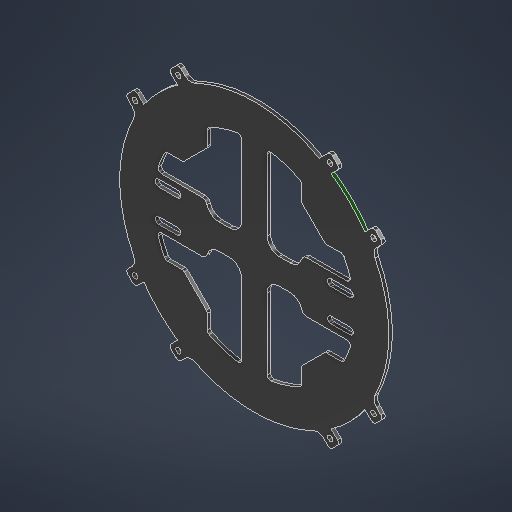
# Autodesk Inventor part: Line Board
Saved by Autodesk Inventor 2026.1 (Build 301233020, 233B)
## iProperties
Created: 2025-11-07
Part Number: Line Board
Material: Generic
Document SubType Name: Modeling
Designer: Bahaa
Density: 1 g/cm^3
Appearance: Glossy - Black
Author: Bahaa
Autodesk Inventor part; units mm, degrees
ref_plane "YZ Plane" through (0, 0, 0) normal (1, 0, 0) x (0, 1, 0)
ref_plane "XZ Plane" through (0, 0, 0) normal (0, 1, 0) x (-1, 0, 0)
ref_plane "XY Plane" through (0, 0, 0) normal (0, 0, 1) x (1, 0, 0)
sketch "Sketch1" plane through (0, 0, 0) normal (0, 1, 0) x (-1, 0, 0)
  circle A0 centre (0, 0) radius 79
  circle A1 centre (0, 0) radius 59
  line L0 (-75, 7.5) -> (75, 7.5)
  line L1 (75, 7.5) -> (75, -7.5)
  line L2 (75, -7.5) -> (-75, -7.5)
  line L3 (-75, -7.5) -> (-75, 7.5)
  line L4 (-75, 7.5) -> (75, -7.5) construction
  line L5 (75, 7.5) -> (-75, -7.5) construction
  line L6 (-7.5, -75) -> (-7.5, 75)
  line L7 (7.5, 75) -> (7.5, -75)
  line L8 (75, -7.5) -> (-75, -7.5)
  line L9 (-75, 7.5) -> (75, 7.5)
  line L10 (7.5, 75) -> (7.5, -75)
  line L11 (-7.5, -75) -> (-7.5, 75)
  line L12 (7.5, 25) -> (-7.5, 25)
  line L13 (-25, 7.5) -> (-25, -7.5)
  line L14 (-7.5, -25) -> (7.5, -25)
  line L15 (25, -7.5) -> (25, 7.5)
  line L16 (25, 25) -> (-25, -25) construction
  line L17 (-25, 25) -> (25, -25) construction
  line L18 (-7.5, 25) -> (-25, 7.5)
  line L19 (25, 7.5) -> (7.5, 25)
  line L20 (25, -7.5) -> (7.5, -25)
  line L21 (-25, -7.5) -> (-7.5, -25)
  line L22 (0, 0) -> (57.2756, -57.2756) construction
  line L23 (57.2756, -57.2756) -> (44.5477, -70.0036) construction
  circle A2 centre (44.5477, -70.0036) radius 1.6
  line L24 (44.5477, -70.0036) -> (47.3762, -67.1751) construction
  line L25 (47.3762, -67.1751) -> (50.2046, -70.0036)
  line L26 (50.2046, -70.0036) -> (44.5477, -64.3467)
  line L27 (44.5477, -64.3467) -> (38.8909, -70.0036) construction
  line L28 (38.8909, -70.0036) -> (44.5477, -75.6604)
  line L29 (44.5477, -75.6604) -> (50.2046, -70.0036)
  line L30 (38.8909, -70.0036) -> (38.0953, -69.208)
  line L31 (44.5477, -64.3467) -> (45.0778, -64.8768)
  circle A3 centre (70.0036, -44.5477) radius 1.6
  line L32 (70.0036, -44.5477) -> (67.1751, -47.3762) construction
  line L33 (67.1751, -47.3762) -> (70.0036, -50.2046)
  line L34 (70.0036, -50.2046) -> (64.3467, -44.5477)
  line L35 (64.3467, -44.5477) -> (70.0036, -38.8909) construction
  line L36 (70.0036, -38.8909) -> (75.6604, -44.5477)
  line L37 (75.6604, -44.5477) -> (70.0036, -50.2046)
  line L38 (70.0036, -38.8909) -> (69.208, -38.0953)
  line L39 (64.3467, -44.5477) -> (64.8768, -45.0778)
  line L40 (64.3467, 44.5477) -> (64.8768, 45.0778)
  line L41 (70.0036, 38.8909) -> (69.208, 38.0953)
  line L42 (64.3467, 44.5477) -> (70.0036, 38.8909) construction
  line L43 (70.0036, 44.5477) -> (67.1751, 47.3762) construction
  circle A4 centre (70.0036, 44.5477) radius 1.6
  line L44 (70.0036, 50.2046) -> (64.3467, 44.5477)
  line L45 (70.0036, 38.8909) -> (75.6604, 44.5477)
  line L46 (75.6604, 44.5477) -> (70.0036, 50.2046)
  line L47 (57.2756, 57.2756) -> (70.0036, 44.5477) construction
  line L48 (67.1751, 47.3762) -> (70.0036, 50.2046)
  line L49 (44.5477, 64.3467) -> (45.0778, 64.8768)
  line L50 (47.3762, 67.1751) -> (50.2046, 70.0036)
  line L51 (50.2046, 70.0036) -> (44.5477, 64.3467)
  line L52 (44.5477, 70.0036) -> (47.3762, 67.1751) construction
  circle A5 centre (44.5477, 70.0036) radius 1.6
  line L53 (44.5477, 75.6604) -> (50.2046, 70.0036)
  line L54 (44.5477, 64.3467) -> (38.8909, 70.0036) construction
  line L55 (38.8909, 70.0036) -> (38.0953, 69.208)
  line L56 (38.8909, 70.0036) -> (44.5477, 75.6604)
  line L57 (-44.5477, 64.3467) -> (-45.0778, 64.8768)
  line L58 (-38.8909, 70.0036) -> (-38.0953, 69.208)
  line L59 (-44.5477, 64.3467) -> (-38.8909, 70.0036) construction
  line L60 (-44.5477, 70.0036) -> (-47.3762, 67.1751) construction
  circle A6 centre (-44.5477, 70.0036) radius 1.6
  line L61 (-50.2046, 70.0036) -> (-44.5477, 64.3467)
  line L62 (-38.8909, 70.0036) -> (-44.5477, 75.6604)
  line L63 (-44.5477, 75.6604) -> (-50.2046, 70.0036)
  line L64 (-57.2756, 57.2756) -> (-44.5477, 70.0036) construction
  line L65 (-47.3762, 67.1751) -> (-50.2046, 70.0036)
  line L66 (-64.3467, 44.5477) -> (-64.8768, 45.0778)
  line L67 (-67.1751, 47.3762) -> (-70.0036, 50.2046)
  line L68 (-70.0036, 50.2046) -> (-64.3467, 44.5477)
  line L69 (-70.0036, 44.5477) -> (-67.1751, 47.3762) construction
  circle A7 centre (-70.0036, 44.5477) radius 1.6
  line L70 (-75.6604, 44.5477) -> (-70.0036, 50.2046)
  line L71 (-64.3467, 44.5477) -> (-70.0036, 38.8909) construction
  line L72 (-70.0036, 38.8909) -> (-69.208, 38.0953)
  line L73 (-70.0036, 38.8909) -> (-75.6604, 44.5477)
  line L74 (-64.3467, -44.5477) -> (-64.8768, -45.0778)
  line L75 (-70.0036, -38.8909) -> (-69.208, -38.0953)
  line L76 (-64.3467, -44.5477) -> (-70.0036, -38.8909) construction
  line L77 (-70.0036, -44.5477) -> (-67.1751, -47.3762) construction
  circle A8 centre (-70.0036, -44.5477) radius 1.6
  line L78 (-70.0036, -50.2046) -> (-64.3467, -44.5477)
  line L79 (-70.0036, -38.8909) -> (-75.6604, -44.5477)
  line L80 (-75.6604, -44.5477) -> (-70.0036, -50.2046)
  line L81 (-57.2756, -57.2756) -> (-70.0036, -44.5477) construction
  line L82 (-67.1751, -47.3762) -> (-70.0036, -50.2046)
  line L83 (-44.5477, -64.3467) -> (-45.0778, -64.8768)
  line L84 (-47.3762, -67.1751) -> (-50.2046, -70.0036)
  line L85 (-50.2046, -70.0036) -> (-44.5477, -64.3467)
  line L86 (-44.5477, -70.0036) -> (-47.3762, -67.1751) construction
  circle A9 centre (-44.5477, -70.0036) radius 1.6
  line L87 (-44.5477, -75.6604) -> (-50.2046, -70.0036)
  line L88 (-44.5477, -64.3467) -> (-38.8909, -70.0036) construction
  line L89 (-38.8909, -70.0036) -> (-38.0953, -69.208)
  line L90 (-38.8909, -70.0036) -> (-44.5477, -75.6604)
  line L91 (55.8614, 55.8614) -> (65.7609, 45.9619) construction
  line L92 (65.7609, 45.9619) -> (65.6902, 45.8912) construction
  line L93 (65.6902, 45.8912) -> (45.8912, 65.6902)
  line L94 (-45.8912, 65.6902) -> (-65.6902, 45.8912)
  line L95 (-65.6902, -45.8912) -> (-45.8912, -65.6902)
  line L96 (45.8912, -65.6902) -> (65.6902, -45.8912)
  line L97 (70.25, -7.5) -> (87.75, -7.5)
  line L98 (87.75, -7.5) -> (87.75, 7.5)
  line L99 (87.75, 7.5) -> (70.25, 7.5)
  line L100 (70.25, 7.5) -> (70.25, -7.5)
  line L101 (70.25, -7.5) -> (87.75, 7.5) construction
  line L102 (87.75, -7.5) -> (70.25, 7.5) construction
  line L103 (0, -7.5) -> (0, 7.5) construction
  line L104 (-70.25, -7.5) -> (-87.75, -7.5)
  line L105 (-87.75, -7.5) -> (-87.75, 7.5)
  line L106 (-87.75, 7.5) -> (-70.25, 7.5)
  line L107 (-70.25, 7.5) -> (-70.25, -7.5)
  line L108 (10, 49) -> (-10, 49)
  line L109 (-10, 49) -> (-10, 59) construction
  line L110 (-10, 59) -> (10, 59) construction
  line L111 (10, 59) -> (10, 49) construction
  line L112 (10, 49) -> (-10, 59) construction
  line L113 (-10, 49) -> (10, 59) construction
  line L114 (10, 49) -> (17.3816, 56.3816)
  line L115 (10, 49) -> (24.951, 49) construction
  line L116 (-10, 49) -> (-17.3816, 56.3816)
  line L117 (-41.7193, 27.5772) -> (-52.1584, 27.5772)
  line L118 (-27.5772, 41.7193) -> (-41.7193, 27.5772)
  line L119 (-27.5772, 41.7193) -> (-27.5772, 52.1584)
  line L120 (-49, -10) -> (-56.3816, -17.3816)
  line L121 (-49, 10) -> (-49, -10)
  line L122 (-49, 10) -> (-56.3816, 17.3816)
  line L123 (-27.5772, -41.7193) -> (-27.5772, -52.1584)
  line L124 (-41.7193, -27.5772) -> (-27.5772, -41.7193)
  line L125 (-41.7193, -27.5772) -> (-52.1584, -27.5772)
  line L126 (10, -49) -> (17.3816, -56.3816)
  line L127 (-10, -49) -> (10, -49)
  line L128 (-10, -49) -> (-17.3816, -56.3816)
  line L129 (41.7193, -27.5772) -> (52.1584, -27.5772)
  line L130 (27.5772, -41.7193) -> (41.7193, -27.5772)
  line L131 (27.5772, -41.7193) -> (27.5772, -52.1584)
  line L132 (49, 10) -> (56.3816, 17.3816)
  line L133 (49, -10) -> (49, 10)
  line L134 (49, -10) -> (56.3816, -17.3816)
  line L135 (27.5772, 41.7193) -> (27.5772, 52.1584)
  line L136 (41.7193, 27.5772) -> (27.5772, 41.7193)
  line L137 (41.7193, 27.5772) -> (52.1584, 27.5772)
  line L138 (28, 15) -> (43, 15)
  line L139 (43, 15) -> (43, -15)
  line L140 (43, -15) -> (28, -15)
  line L141 (28, -15) -> (28, 15)
  line L142 (28, 15) -> (43, -15) construction
  line L143 (43, 15) -> (28, -15) construction
  line L144 (49, 0) -> (25, 0) construction
  line L145 (-25, -7.5) -> (-25, 7.5)
  line L146 (-28, 15) -> (-43, 15)
  line L147 (-43, 15) -> (-43, -15)
  line L148 (-43, -15) -> (-28, -15)
  line L149 (-28, -15) -> (-28, 15)
  line L150 (-28, 15) -> (-43, -15) construction
  line L151 (-43, 15) -> (-28, -15) construction
  line L152 (-43, -15) -> (-57.8684, -15)
  line L153 (-57.8684, -15) -> (-57.8684, -11.5)
  line L154 (-57.8684, -11.5) -> (-43, -11.5)
  line L155 (-43, -11.5) -> (-43, -15)
  line L156 (-43, 15) -> (-57.8684, 15)
  line L157 (-57.8684, 15) -> (-57.8684, 11.5)
  line L158 (-57.8684, 11.5) -> (-43, 11.5)
  line L159 (43, -15) -> (57.8684, -15)
  line L160 (57.8684, -15) -> (57.8684, -11.5)
  line L161 (57.8684, -11.5) -> (43, -11.5)
  line L162 (43, -11.5) -> (43, -15)
  line L163 (43, 15) -> (57.8684, 15)
  line L164 (57.8684, 15) -> (57.8684, 11.5)
  line L165 (57.8684, 11.5) -> (43, 11.5)
  point P0 (-58.5214, 7.5)
  point P1 (-7.5, 58.5214)
  point P2 (-7.5, 25)
  point P3 (-25, 7.5)
  point P4 (-58.5214, -7.5)
  point P5 (-25, -7.5)
  point P6 (-7.5, -25)
  point P7 (-7.5, -58.5214)
  point P8 (-74.6241, 7.5)
  point P9 (-74.6241, -7.5)
  point P10 (-69.208, -38.0953)
  point P11 (-64.8768, -45.0778)
  point P12 (-45.0778, -64.8768)
  point P13 (-38.0953, -69.208)
  point P14 (64.8768, -45.0778)
  point P15 (69.208, -38.0953)
  point P16 (74.6241, -7.5)
  point P17 (74.6241, 7.5)
  point P18 (69.208, 38.0953)
  point P19 (64.8768, 45.0778)
  point P20 (45.0778, 64.8768)
  point P21 (38.0953, 69.208)
  point P22 (-38.0953, 69.208)
  point P23 (-45.0778, 64.8768)
  point P24 (-64.8768, 45.0778)
  point P25 (-69.208, 38.0953)
  point P26 (58.5214, -7.5)
  point P27 (7.5, -58.5214)
  point P28 (7.5, -25)
  point P29 (25, -7.5)
  point P30 (58.5214, 7.5)
  point P31 (25, 7.5)
  point P32 (7.5, 25)
  point P33 (7.5, 58.5214)
  point P34 (-38.8202, 69.9329)
  point P35 (-69.9329, 38.8202)
  point P36 (-69.9329, -38.8202)
  point P37 (-38.8202, -69.9329)
  point P38 (38.8202, -69.9329)
  point P39 (69.9329, -38.8202)
  point P40 (-65.6902, -45.8912)
  point P41 (-58.6005, -52.9809)
  point P42 (-45.8912, -65.6902)
  point P43 (-52.9809, -58.6005)
  point P44 (-45.8912, 65.6902)
  point P45 (-52.9809, 58.6005)
  point P46 (45.8912, -65.6902)
  point P47 (52.9809, -58.6005)
  point P48 (58.6005, -52.9809)
  point P49 (58.6005, 52.9809)
  point P50 (65.6902, 45.8912)
  point P51 (52.9809, 58.6005)
  point P52 (-58.6005, 52.9809)
  point P53 (-65.6902, 45.8912)
  point P54 (79, 0)
  point P55 (78.6432, 7.5)
  point P56 (78.6432, -7.5)
  point P57 (-78.6432, -7.5)
  point P58 (-78.6432, 7.5)
  point P59 (0, 0)
  point P60 (-7.5, 7.5)
  point P61 (-7.5, -7.5)
  point P62 (7.5, -7.5)
  point P63 (7.5, 7.5)
  point P64 (0, 54)
  point P65 (-52.1584, -27.5772)
  point P66 (-27.5772, -52.1584)
  point P67 (27.5772, -52.1584)
  point P68 (52.1584, -27.5772)
  point P69 (27.5772, 52.1584)
  point P70 (-27.5772, 52.1584)
  point P71 (-52.1584, 27.5772)
  point P72 (45.0778, 64.8768)
  point P73 (64.8768, -45.0778)
  point P74 (-45.0778, -64.8768)
  point P75 (-64.8768, 45.0778)
  point P76 (35.5, 0)
  point P77 (28, 7.5)
  point P78 (43, 7.5)
  point P79 (43, -7.5)
  point P80 (28, -7.5)
  point P81 (-35.5, 0)
  point P82 (-25, 0)
  point P83 (-43, 7.5)
  point P84 (-28, 7.5)
  point P85 (-28, -7.5)
  point P86 (-43, -7.5)
  point P87 (-57.0614, 15)
  point P88 (-57.0614, -15)
  point P89 (57.0614, 15)
  point P90 (57.0614, -15)
  dimension "d0" = 158
  dimension "d1" = 20
  dimension "d2" = 150
  dimension "d3" = 15
  dimension "d6" = 360
  dimension "d8" = 50
  dimension "d9" = 50
  dimension "d10" = 17.5
  dimension "d11" = 17.5
  dimension "d12" = 17.5
  dimension "d13" = 17.5
  dimension "d14" = 17.5
  dimension "d15" = 17.5
  dimension "d16" = 17.5
  dimension "d17" = 17.5
  dimension "d18" = 81
  dimension "d19" = 18
  dimension "d20" = 3.2
  dimension "d23" = 4
  dimension "d24" = 4
  dimension "d25" = 8
  dimension "d26" = 8
  dimension "d27" = 8
  dimension "d30" = 360
  dimension "d36" = 0.1
  dimension "d39" = 360
  dimension "d50" = 17.5
  dimension "d51" = 15
  dimension "d52" = 70.25
  dimension "d68" = 10
  dimension "d69" = 20
  dimension "d70" = 0
  dimension "d71" = 0
  dimension "d73" = 45
  dimension "d76" = 360
  dimension "d79" = 30
  dimension "d80" = 28
  dimension "d81" = 15
  dimension "d83" = 30
  dimension "d84" = 15
  dimension "d85" = 4
  dimension "d86" = 4
  constraints: 332 end point, 24 point on line, 22 symmetric about line, 18 parallel, 17 midpoint, 14 perpendicular, 9 coincident, 9 horizontal, 8 centre point, 261 other
  measures "d2" distance of L1.end L2.end
  measures "d3" distance of L0.end L1.end
  measures "d8" distance of L17.end L16.end
  measures "d9" distance of L16.end L17.start
  measures "d10" distance of L12.end L17.start
  measures "d11" distance of L13.start L17.start
  measures "d12" distance of L15.end L16.start
  measures "d13" distance of L12.start L16.start
  measures "d14" distance of L15.start L17.end
  measures "d15" distance of L14.end L17.end
  measures "d16" distance of L13.end L16.end
  measures "d17" distance of L14.start L16.end
  measures "d18" distance of L22.start L22.end
  measures "d19" distance of L22.end L23.end
  measures "d20" diameter of A2
  measures "d23" distance of L24.start L24.end
  measures "d24" distance of L24.end L25.end
  measures "d25" distance of L25.end L26.end
  measures "d26" distance of L27.end L26.end
  measures "d27" distance between parallel lines of L30 L31
  measures "d36" distance of L91.end L92.end
  measures "d50" distance of L99.end L98.end
  measures "d51" distance of L98.end L97.end
  measures "d52" distance from line of L22.start L100
  measures "d68" distance of L108.end L109.end
  measures "d69" distance of L108.start L108.end
  measures "d70" vertical extent of L110
  measures "d71" horizontal distance of L22.start point (0, 54)
  measures "d73" angle of L115 L114
  measures "d79" distance of L140.end L138.start
  measures "d80" distance from line of L22.start L141
  measures "d81" distance of L139.end L140.end
  measures "d83" distance of L146.end L147.end
  measures "d84" distance of L147.end L148.end
  measures "d85" distance between parallel lines of L8 L154
  measures "d86" distance between parallel lines of L8 L161
extrude "Extrusion1" add sketch "Sketch1" along normal blind 2 contours A0 L99 L0 A1 L164 L163 L156 L157 L106 L94 L93 | A0 L44 L46 L45 L41 | A0 L97 L1 L99 | L93 A0 | L1 L2 L100 L0 | A0 L96 L95 L104 L2 A1 L153 L152 L159 L160 L97 | L100 L2 A1 L0 | A0 L55 L56 L53 L50 L51 | L38 L36 L37 L33 L34 A0 | A1 L2 L133 L0 | L165 L132 L163 A1 | A1 L163 L164 | L133 L2 L139 L0 | A0 L61 L63 L62 L58 | A0 L96 | L165 L139 L163 L132 | L139 L2 L141 L0 | L0 L141 L138 L139 | L160 L159 A1 | A1 L159 L134 L161 | L141 L2 L15 L0 | L139 L140 L141 L2 | L134 L159 L139 L161 | L94 A0 | L26 L25 L29 L28 L30 A0 | L137 L136 L135 A1 | L15 L2 L7 L0 | L7 L2 L6 L0 | L0 L6 L12 L7 | L12 L6 L108 L7 | A1 L131 L130 L129 | A0 L72 L73 L70 L67 L68 | L89 L90 L87 L84 L85 A0 | L6 L2 L13 L0 | L7 L14 L6 L2 | L7 L127 L6 L14 | L108 L6 A1 L7 | L13 L2 L149 L0 | L7 A1 L6 L127 | L106 L3 L104 A0 | A0 L95 | L149 L2 L147 L0 | L0 L147 L146 L149 | L0 L107 L2 L3 | L147 L2 L121 L0 | L149 L148 L147 L2 | A0 L78 L80 L79 L75 | L0 A1 L2 L107 | L119 L118 L117 A1 | L121 L2 A1 L0 | L158 L122 L156 L147 | L158 A1 L156 L122 | L147 L152 L120 L154 | A1 L125 L124 L123 | L157 L156 A1 | L120 L152 A1 L154 | A1 L152 L153
fillet "Fillet1" radius 2 56 edges at (-75.6604, 1, 44.5477) (-70.0036, 1, 50.2046) (-44.5477, 1, 75.6604) (-50.2046, 1, 70.0036) (44.5477, 1, 75.6604) (50.2046, 1, 70.0036) (70.0036, 1, 50.2046) (75.6604, 1, 44.5477) (75.6604, 1, -44.5477) (70.0036, 1, -50.2046) (50.2046, 1, -70.0036) (44.5477, 1, -75.6604) (-50.2046, 1, -70.0036) (-44.5477, 1, -75.6604) (-75.6604, 1, -44.5477) (-70.0036, 1, -50.2046) (-7.5, 1, 58.5214) (-58.5214, 1, 7.5) (-58.5214, 1, -7.5) (-7.5, 1, -58.5214) (7.5, 1, -58.5214) (58.5214, 1, -7.5) (58.5214, 1, 7.5) (7.5, 1, 58.5214) (27.5772, 1, 41.7193) (27.5772, 1, 52.1584) (41.7193, 1, 27.5772) (52.1584, 1, 27.5772) (52.1584, 1, -27.5772) (41.7193, 1, -27.5772) (27.5772, 1, -41.7193) (27.5772, 1, -52.1584) (-27.5772, 1, -52.1584) (-27.5772, 1, -41.7193) (-41.7193, 1, -27.5772) (-52.1584, 1, -27.5772) (-52.1584, 1, 27.5772) (-41.7193, 1, 27.5772) (-27.5772, 1, 41.7193) (-27.5772, 1, 52.1584) (57.8684, 1, 11.5) (43, 1, 7.5) (43, 1, 11.5) (43, 1, -11.5) (43, 1, -7.5) (57.8684, 1, -11.5) (-43, 1, -11.5) (-57.8684, 1, -11.5) (-43, 1, -7.5) (-43, 1, 7.5) (-43, 1, 11.5) (-57.8684, 1, 11.5) (-57.0614, 1, -15) (-57.0614, 1, 15) (57.0614, 1, 15) (57.0614, 1, -15)
fillet "Fillet2" radius 5 7 edges at (69.208, 1, 38.0953) (69.208, 1, -38.0953) (38.0953, 1, -69.208) (-38.0953, 1, -69.208) (-69.208, 1, -38.0953) (-69.208, 1, 38.0953) (-38.0953, 1, 69.208)
sketch "Sketch2" plane through (0, 2, 0) normal (0, -1, 0) x (1, 0, 0)
  line L0 (-65, -15) -> (65, -15) construction
  line L1 (65, -15) -> (65, 15) construction
  line L2 (65, 15) -> (-65, 15) construction
  line L3 (-65, 15) -> (-65, -15) construction
  line L4 (-65, -15) -> (65, 15) construction
  line L5 (65, -15) -> (-65, 15) construction
  line L6 (0, 15) -> (0, 12) construction
  line L7 (0, 0) -> (65, 0) construction
  circle A0 centre (0, 12) radius 1.35
  circle A1 centre (0, 12) radius 2.55
  circle A2 centre (0, -12) radius 1.35
  circle A3 centre (0, -12) radius 2.55
  dimension "d41" = 130
  dimension "d42" = 30
  dimension "d43" = 3
  dimension "d44" = 2.7
  dimension "d45" = 5.1
  dimension "d46" = 2.7
  dimension "d47" = 5.1
  constraints: 16 end point, 5 coincident, 4 centre point, 4 midpoint, 2 parallel, 1 horizontal, 1 perpendicular, 1 symmetric about line, 1 vertical
  measures "d41" distance of L2.end L1.end
  measures "d42" distance of L1.end L0.end
  measures "d43" distance of L6.start L6.end
  measures "d44" diameter of A0
  measures "d45" diameter of A1
  measures "d46" diameter of A2
  measures "d47" diameter of A3
extrude "Extrusion2" [suppressed]
fillet "Fillet3" radius 7 8 edges at (7.5, 1, -7.5) (-7.5, 1, -7.5) (-7.5, 1, 7.5) (7.5, 1, 7.5) (-28, 1, 7.5) (-28, 1, -7.5) (28, 1, -7.5) (28, 1, 7.5)
fillet "Fillet4" radius 3 4 edges at (-28, 1, -15) (-28, 1, 15) (28, 1, 15) (28, 1, -15)
equation "\"d11\" = d10"
equation "\"d12\" = d10"
equation "\"d13\" = d12"
equation "\"d14\" = d10"
equation "\"d15\" = d14"
equation "\"d16\" = d10"
equation "\"d17\" = d16"
equation "\"d24\" = d23"
equation "\"d25\" = 2 * d23"
equation "\"d27\" = 2 * d23"
body "Solid1"
